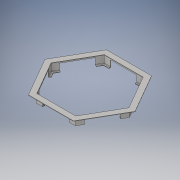
# Autodesk Inventor part: KiloHexiThing
Saved by Autodesk Inventor 2016 (Build 200138000, 138)
## iProperties
Created: 2016-05-26
Part Number: KiloHexiThing
Material: Generic
Document SubType Name: Modeling
Designer: jllonsfo
Density: 1 g/cm^3
Appearance: Default
Author: jllonsfo
Autodesk Inventor part; units mm, degrees
ref_plane "YZ Plane" through (0, 0, 0) normal (1, 0, 0) x (0, 1, 0)
ref_plane "XZ Plane" through (0, 0, 0) normal (0, 1, 0) x (-1, 0, 0)
ref_plane "XY Plane" through (0, 0, 0) normal (0, 0, 1) x (1, 0, 0)
sketch "Sketch1" plane through (0, 0, 0) normal (0, 1, 0) x (-1, 0, 0)
  line L0 (89.8, 0) -> (44.9, -77.7691)
  line L1 (44.9, -77.7691) -> (-44.9, -77.7691)
  line L2 (-44.9, -77.7691) -> (-89.8, 0)
  line L3 (-89.8, 0) -> (-44.9, 77.7691)
  line L4 (-44.9, 77.7691) -> (44.9, 77.7691)
  line L5 (44.9, 77.7691) -> (89.8, 0)
  line L6 (88.6453, 0) -> (44.3226, -76.7691)
  line L7 (44.3226, -76.7691) -> (-44.3226, -76.7691)
  line L8 (-44.3226, -76.7691) -> (-88.6453, 0)
  line L9 (-88.6453, 0) -> (-44.3226, 76.7691)
  line L10 (-44.3226, 76.7691) -> (44.3226, 76.7691)
  line L11 (44.3226, 76.7691) -> (88.6453, 0)
  point P0 (0, 0)
  point P1 (0, 0)
  dimension "d0" = 89.8
  dimension "d1" = 1
  constraints: 24 end point, 1 coincident, 18 other
  measures "d0" distance of L0.start L4.end
  measures "d1" distance between parallel lines of L5 L11
extrude "Extrusion1" add sketch "Sketch1" along normal blind 17.48
sketch "Sketch10" plane through (0, 0, 0) normal (0, -1, 0) x (1, 0, 0)
  line L0 (-89.8, 0) -> (-44.9, -77.7691) projected
  line L1 (-89.8, 0) -> (-44.9, 77.7691)
  line L2 (-44.9, 77.7691) -> (44.9, 77.7691)
  line L3 (44.9, 77.7691) -> (89.8, 0)
  line L4 (89.8, 0) -> (44.9, -77.7691)
  line L5 (44.9, -77.7691) -> (-44.9, -77.7691)
  line L6 (-44.9, -77.7691) -> (-89.8, 0)
  line L7 (-84.0265, 0) -> (-42.0132, 72.7691)
  line L8 (-42.0132, 72.7691) -> (42.0132, 72.7691)
  line L9 (42.0132, 72.7691) -> (84.0265, 0)
  line L10 (84.0265, 0) -> (42.0132, -72.7691)
  line L11 (42.0132, -72.7691) -> (-42.0132, -72.7691)
  line L12 (-42.0132, -72.7691) -> (-84.0265, 0)
  point P0 (0, 0)
  point P1 (0, 0)
  point P2 (-82.35, -12.9038)
  point P3 (0, 0)
  dimension "d24" = 5
  constraints: 24 end point, 2 coincident, 26 other
  measures "d24" distance between parallel lines of L6 L12
extrude "Extrusion5" add sketch "Sketch10" against normal blind 1 separate body
sketch "Sketch9" plane through (0, 17.48, 0) normal (0, 1, 0) x (1, 0, 0)
  line L0 (102.5, 0) -> (51.25, -88.7676)
  line L1 (51.25, -88.7676) -> (-51.25, -88.7676)
  line L2 (-51.25, -88.7676) -> (-102.5, 0)
  line L3 (-102.5, 0) -> (-51.25, 88.7676)
  line L4 (-51.25, 88.7676) -> (51.25, 88.7676)
  line L5 (51.25, 88.7676) -> (102.5, 0)
  line L6 (88.6436, 0) -> (44.3218, -76.7676)
  line L7 (44.3218, -76.7676) -> (-44.3218, -76.7676)
  line L8 (-44.3218, -76.7676) -> (-88.6436, 0)
  line L9 (-88.6436, 0) -> (-44.3218, 76.7676)
  line L10 (-44.3218, 76.7676) -> (44.3218, 76.7676)
  line L11 (44.3218, 76.7676) -> (88.6436, 0)
  point P0 (0, 0)
  point P1 (0, 0)
  point P2 (0, 0)
  dimension "d20" = 205
  dimension "d21" = 12
  constraints: 24 end point, 2 coincident, 26 other
  measures "d20" distance of L0.start L2.end
  measures "d21" distance between parallel lines of L1 L7
extrude "Extrusion4" add sketch "Sketch9" along normal blind 1 separate body
combine bodies "Combine1" operation type add bodies to combine 1 2
combine bodies "Combine2" operation type add bodies to combine 1 3
fillet "Fillet3" radius 1 6 edges at (67.35, 17.48, -38.8845) (0, 17.48, -77.7691) (-67.35, 17.48, -38.8845) (-67.35, 17.48, 38.8845) (0, 17.48, 77.7691) (67.35, 17.48, 38.8845)
fillet "Fillet4" radius 1 6 edges at (0, 1, 76.7691) (66.484, 1, 38.3845) (-66.484, 1, 38.3845) (0, 1, -76.7691) (-66.484, 1, -38.3845) (66.484, 1, -38.3845)
sketch "Sketch13" plane through (-44.9, 0, -77.7691) normal (0, -1, 0) x (1, 0, 0)
  line L0 (0.5774, 1) -> (89.2226, 1) projected
  line L1 (44.9, -22.7956) -> (14.9, -22.7956)
  line L2 (14.9, -22.7956) -> (14.9, 21.7864)
  line L3 (14.9, 21.7864) -> (74.9, 21.7864)
  line L4 (74.9, 21.7864) -> (74.9, -22.7956)
  line L5 (74.9, -22.7956) -> (44.9, -22.7956)
  line L6 (116.9916, 1.506) -> (78.3824, 23.797)
  line L7 (131.9916, 27.4867) -> (116.9916, 1.506)
  line L8 (108.3824, 75.7585) -> (146.9916, 53.4675)
  line L9 (146.9916, 53.4675) -> (131.9916, 27.4867)
  line L10 (78.3824, 23.797) -> (108.3824, 75.7585)
  line L11 (146.9916, 102.0707) -> (108.3824, 79.7797)
  line L12 (131.9916, 128.0514) -> (146.9916, 102.0707)
  line L13 (78.3824, 131.7412) -> (116.9916, 154.0322)
  line L14 (116.9916, 154.0322) -> (131.9916, 128.0514)
  line L15 (108.3824, 79.7797) -> (78.3824, 131.7412)
  line L16 (74.9, 178.3338) -> (74.9, 133.7518)
  line L17 (44.9, 178.3338) -> (74.9, 178.3338)
  line L18 (14.9, 133.7518) -> (14.9, 178.3338)
  line L19 (14.9, 178.3338) -> (44.9, 178.3338)
  line L20 (74.9, 133.7518) -> (14.9, 133.7518)
  line L21 (-27.1916, 154.0322) -> (11.4176, 131.7412)
  line L22 (-42.1916, 128.0514) -> (-27.1916, 154.0322)
  line L23 (-18.5824, 79.7797) -> (-57.1916, 102.0707)
  line L24 (-57.1916, 102.0707) -> (-42.1916, 128.0514)
  line L25 (11.4176, 131.7412) -> (-18.5824, 79.7797)
  line L26 (-57.1916, 53.4675) -> (-18.5824, 75.7585)
  line L27 (-42.1916, 27.4867) -> (-57.1916, 53.4675)
  line L28 (11.4176, 23.797) -> (-27.1916, 1.506)
  line L29 (-27.1916, 1.506) -> (-42.1916, 27.4867)
  line L30 (-18.5824, 75.7585) -> (11.4176, 23.797)
  point P0 (44.9, 77.7691)
  dimension "d28" = 60
  dimension "d31" = 360
  constraints: 60 end point, 6 point on line, 4 perpendicular, 61 other
  measures "d28" distance of L2.end L3.end
extrude "Extrusion6" cut sketch "Sketch13" against normal blind 15.2875 bodies 1
body "Solid1"
